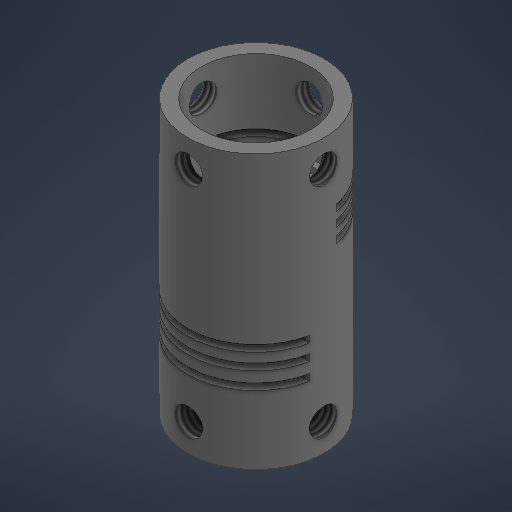
# Autodesk Inventor part: coupler
Saved by Autodesk Inventor 2026.2 (Build 302298010, 298A)
## iProperties
Created: 2026-04-14
Part Number: coupler
Material: Generic
Document SubType Name: Modeling
Designer: yasser
Density: 1 g/cm^3
Appearance: Default
Author: yasser
## iProperties of the stored document coupler_3DPrint.ipt
Created: 2026-04-14
Part Number: coupler_3DPrint
Material: Generic
Document SubType Name: Modeling
Designer: yasser
Density: 1 g/cm^3
Appearance: Default
Author: yasser
Autodesk Inventor part; units mm, degrees
ref_plane "XZ Plane" through (0, 0, 0) normal (0, 1, 0) x (-1, 0, 0)
sketch "Sketch1" plane through (0, 0, 0) normal (0, 1, 0) x (-1, 0, 0)
  circle A0 centre (0, 0) radius 5
  dimension "d0" = 10
  constraints: 1 centre point, 1 coincident
  measures "d0" diameter of A0
extrude "Extrusion1" add sketch "Sketch1" along normal blind 20
sketch "Sketch2" plane through (0, 20, 0) normal (0, 1, 0) x (1, 0, 0)
  circle A0 centre (0, 0) radius 4
  dimension "d3" = 8
  constraints: 1 centre point, 1 coincident
  measures "d3" diameter of A0
extrude "Extrusion2" cut sketch "Sketch2" against normal blind 10
sketch "Sketch3" plane through (0, 0, 0) normal (0, -1, 0) x (1, 0, 0)
  circle A0 centre (0, 0) radius 3
  dimension "d6" = 6
  constraints: 1 centre point, 1 coincident
  measures "d6" diameter of A0
extrude "Extrusion3" cut sketch "Sketch3" against normal blind 10
ref_plane "Work Plane1" through (5, 0, 0) normal (1, 0, 0) x (0, 1, 0)
sketch "Sketch4" plane through (5, 0, 0) normal (1, 0, 0) x (0, 1, 0)
  circle A0 centre (18, 0) radius 1
  circle A1 centre (2, 0) radius 1
  line L0 (20, -5) -> (20, 5) projected
  line L1 (0, -5) -> (20, -5) projected
  line L2 (15.2461, -5) -> (14.7461, -5)
  line L3 (14.7461, -5) -> (14.7461, -1)
  line L4 (14.7461, -1) -> (15.2461, -1)
  line L5 (15.2461, -1) -> (15.2461, -5)
  line L6 (0, -5) -> (20, -5) projected
  line L7 (14.2461, -5) -> (13.7461, -5)
  line L8 (13.7461, -5) -> (13.7461, -1)
  line L9 (13.7461, -1) -> (14.2461, -1)
  line L10 (14.2461, -1) -> (14.2461, -5)
  line L11 (0, -5) -> (20, -5) projected
  line L12 (13.2461, -5) -> (12.7461, -5)
  line L13 (12.7461, -5) -> (12.7461, -1)
  line L14 (12.7461, -1) -> (13.2461, -1)
  line L15 (13.2461, -1) -> (13.2461, -5)
  line L16 (0, 5) -> (20, 5) projected
  line L17 (0, 2.8) -> (10, 2.8) projected
  line L18 (0, 5) -> (20, 5) projected
  line L19 (5, 5) -> (5.5, 5)
  line L20 (5.5, 5) -> (5.5, 1)
  line L21 (5.5, 1) -> (5, 1)
  line L22 (5, 1) -> (5, 5)
  line L23 (6.2542, 5) -> (6.7542, 5)
  line L24 (6.7542, 5) -> (6.7542, 1)
  line L25 (6.7542, 1) -> (6.2542, 1)
  line L26 (6.2542, 1) -> (6.2542, 5)
  line L27 (7.4248, 5) -> (7.9248, 5)
  line L28 (7.9248, 5) -> (7.9248, 1)
  line L29 (7.9248, 1) -> (7.4248, 1)
  line L30 (7.4248, 1) -> (7.4248, 5)
  point P0 (0, 0)
  point P1 (0, 3)
  point P2 (10, 3)
  point P3 (0, 3)
  point P4 (10, 3)
  dimension "d10" = 2
  dimension "d11" = 2
  dimension "d12" = 2
  dimension "d13" = 2
  dimension "d23" = 0.5
  dimension "d26" = 0.5
  dimension "d27" = 0.5
  dimension "d28" = 4
  dimension "d31" = 0.5
  constraints: 48 end point, 12 parallel, 10 point on line, 6 horizontal, 6 perpendicular, 4 equal length, 2 centre point, 1 other
  measures "d10" diameter of A0
  measures "d11" diameter of A1
  measures "d12" distance from line of A0.centre L0
  measures "d13" distance of point (0, 0) A1.centre
  measures "d23" distance of L3.end L4.end
  measures "d26" distance of L7.start L2.end
  measures "d27" distance of L12.start L7.end
  measures "d28" distance of L12.end L13.end
  measures "d31" distance of L28.end L29.end
extrude "Extrusion4" cut sketch "Sketch4" against normal blind 10 contours A0 | A1 | L28 L17 L30 L16 | L1 L13 L14 L15 | L1 L8 L9 L10 | L1 L3 L4 L5 | L28 L29 L30 L17 | L24 L17 L26 L16 | L24 L25 L26 L17 | L20 L17 L22 L16 | L20 L21 L22 L17
ref_plane "Work Plane2" through (0, 0, 5) normal (0, 0, 1) x (1, 0, 0)
sketch "Sketch5" plane through (0, 0, 5) normal (0, 0, 1) x (1, 0, 0)
  circle A0 centre (0, 18) radius 1
  circle A1 centre (0, 2) radius 1
  line L0 (5, 20) -> (-5, 20) projected
  point P0 (0, 0)
  dimension "d17" = 2
  dimension "d18" = 2
  dimension "d19" = 2
  dimension "d20" = 2
  constraints: 2 centre point
  measures "d17" diameter of A0
  measures "d18" diameter of A1
  measures "d19" distance from line of A0.centre L0
  measures "d20" distance of point (0, 0) A1.centre
extrude "Extrusion5" cut sketch "Sketch5" against normal blind 10
thread "Thread1" size "M2x0.4" class "6H" standard "ANSI Metric M Profile" full length
thread "Thread2" size "M2x0.4" class "6H" standard "ANSI Metric M Profile" full length
thread "Thread3" size "M2x0.4" class "6H" standard "ANSI Metric M Profile" full length
thread "Thread4" size "M2x0.4" class "6H" standard "ANSI Metric M Profile" full length
body "Solid1"
